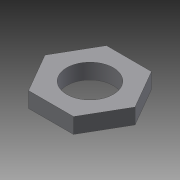
# Autodesk Inventor part: 3-16in_1-16in_nut(num2)
Saved by Autodesk Inventor 2015 (Build 190159000, 159)
## iProperties
Created: 2017-01-13
Part Number: 3-16in_1-16in_nut(num2)
Material: Generic
Document SubType Name: Modeling
Designer: Guy
Density: 1 g/cm^3
Appearance: Default
Mass: 0.0597086 g
Surface Area: 1.42969 cm^2
Volume: 0.0597086 cm^3
Author: Guy
Autodesk Inventor part; units mm, degrees
ref_plane "YZ Plane" through (0, 0, 0) normal (1, 0, 0) x (0, 1, 0)
ref_plane "XZ Plane" through (0, 0, 0) normal (0, 1, 0) x (-1, 0, 0)
ref_plane "XY Plane" through (0, 0, 0) normal (0, 0, 1) x (1, 0, 0)
sketch "Sketch1" plane through (0, 0, 0) normal (0, 0, 1) x (1, 0, 0)
  circle A0 centre (0, 0) radius 2.3813
  line L0 (-2.3094, -4) -> (-4.6188, 0)
  circle A1 centre (0, 0) radius 4
  line L1 (0, 0) -> (21.1791, 0)
  line L2 (0, 0) -> (-22.2603, 0)
  line L3 (-2.3094, -4) -> (2.3094, -4)
  line L4 (2.3094, -4) -> (4.6188, 0)
  line L5 (4.6188, 0) -> (2.3094, 4)
  line L6 (2.3094, 4) -> (-2.3094, 4)
  line L7 (-2.3094, 4) -> (-4.6188, 0)
  dimension "d0" = 4.7625
  dimension "d1" = 8
  dimension "d2" = 120
  constraints: 16 end point, 6 tangent, 3 horizontal, 2 centre point, 2 coincident, 2 parallel, 2 point on line
  measures "d0" diameter of A0
  measures "d1" diameter of A1
  measures "d2" angle of L6 L5
extrude "Extrusion2" add sketch "Sketch1" along normal blind 1.5875
sketch "Sketch2" plane through (0, 0, 0) normal (0, 0, -1) x (-1, 0, 0)
  circle A0 centre (0, 0) radius 2.3813
  dimension "d7" = 4.7625
  constraints: 1 centre point, 1 coincident
  measures "d7" diameter of A0
extrude "Extrusion3" cut sketch "Sketch2" against normal through all
equation "\"d8\" = d7"
body "Solid2"
